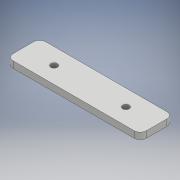
# Autodesk Inventor part: shovel_side
Saved by Autodesk Inventor 2017.2 (Build 212233000, 233)
## iProperties
Created: 2017-09-14
Part Number: shovel_side
Material: Generic
Document SubType Name: Modeling
Designer: Nic
Density: 1 g/cm^3
Appearance: Default
Author: Nic
Autodesk Inventor part; units mm, degrees
ref_plane "YZ Plane" through (0, 0, 0) normal (1, 0, 0) x (0, 1, 0)
ref_plane "XZ Plane" through (0, 0, 0) normal (0, 1, 0) x (-1, 0, 0)
ref_plane "XY Plane" through (0, 0, 0) normal (0, 0, 1) x (1, 0, 0)
sketch "Sketch1" plane through (0, 0, 0) normal (0, 0, 1) x (1, 0, 0)
  line L0 (-32.5, -5) -> (-32.5, 5)
  line L1 (-29.5, 8) -> (29.5, 8)
  line L2 (32.5, -5) -> (32.5, 5)
  line L3 (-29.5, -8) -> (29.5, -8)
  arc A0 (-29.5, 8) -> (-32.5, 5) centre (-29.5, 5) ccw
  arc A1 (-32.5, -5) -> (-29.5, -8) centre (-29.5, -5) ccw
  arc A2 (32.5, 5) -> (29.5, 8) centre (29.5, 5) ccw
  arc A3 (29.5, -8) -> (32.5, -5) centre (29.5, -5) ccw
  line L4 (0, 8) -> (0, -8) construction
  line L5 (-32.5, 0) -> (32.5, 0) construction
  circle A4 centre (-17.5, 0) radius 1.6
  circle A5 centre (17.5, 0) radius 1.6
  point P0 (-32.5, -8)
  point P1 (-32.5, 8)
  point P2 (32.5, -2.2581)
  point P3 (0, 0)
  point P4 (0, 0)
  dimension "d16" = 3
  dimension "d17" = 16
  dimension "d18" = 65
  dimension "d19" = 35
  dimension "d20" = 3.2
  constraints: 12 end point, 8 point on circle, 8 tangent, 7 point on line, 6 centre point, 5 midpoint, 3 equal radius, 1 coincident, 1 horizontal, 1 perpendicular, 1 vertical, 1 other
  measures "d16" radius of A0
  measures "d17" distance between parallel lines of L3 L1
  measures "d18" distance between parallel lines of L2 L0
  measures "d19" distance of A5.centre A4.centre
  measures "d20" diameter of A4
extrude "Extrusion1" add sketch "Sketch1" along normal blind 3.175
body "Solid1"
